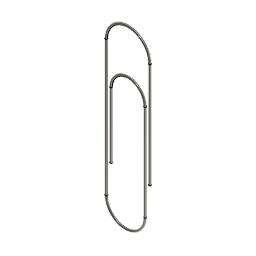
Sketch16_Final v4 (Autodesk Fusion 360 design; units mm, degrees)
Autodesk Fusion 360 part; units mm, degrees
sketch "Sketch1" plane through (0, 0, 0) normal (0, 1, 0) x (1, 0, 0)
  line L0 (5, 0) -> (4.9999, -24)
  line L1 (-4.9998, -24.05) -> (-5, 6.95)
  line L2 (3.9, 7) -> (3.9, -15)
  line L3 (-3.9, -15) -> (-3.9, 0)
  arc A0 (-3.9, -15) -> (3.9, -15) centre (0, -15) ccw
  line L4 (-5, 6.95) -> (-5, 7)
  arc A1 (-4.9998, -24.05) -> (4.9999, -24) centre (-0.0001, -24) ccw
  arc A2 (3.9, 7) -> (-5, 7) centre (-0.55, 7) ccw
  dimension "d29" = 24
  dimension "d30" = 31
  dimension "d31" = 22
  dimension "d32" = 15
  constraint coincident L1 L4.end
  measures "d29" distance of L0.start L0.end
  measures "d30" distance of L1.start L1.end
  measures "d31" distance of L2.end L2.start
  measures "d32" distance of L3.end L3.start
sketch "Sketch4" plane through (0, 0, 0) normal (0, 0, 1) x (1, 0, 0)
  circle A0 centre (5, 0) radius 0.25
  dimension "d35" = 5
  dimension "d36" = 0.5
  measures "d35" distance of origin A0.centre
  measures "d36" diameter of A0
sweep "Sweep2" add profiles "Sketch4" path "Sketch1" along L0 A1 L1 L4 A2 L2 A0 L3 section 1
sketch "Sketch2" plane through (0, 0, 0) normal (0, 0, 1) x (1, 0, 0)
  circle A0 centre (5, 0) radius 0.25
  dimension "d22" = 0.5
  measures "d22" diameter of A0
sweep "Sweep1" [suppressed]
